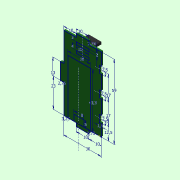
# Autodesk Inventor part: Motherboard_dummy
Saved by Autodesk Inventor 2015 (Build 190159000, 159)
## iProperties
Created: 2014-12-25
Part Number: Motherboard_dummy
Material: ABS Plastic
Document SubType Name: Modeling
Designer: Openlab
Density: 1.06 g/cm^3
Appearance: Smooth - Dark Forest Green
Mass: 9.08054 g
Surface Area: 59.127 cm^2
Volume: 8.56654 cm^3
Author: Openlab
Autodesk Inventor part; units mm, degrees
ref_plane "YZ Plane" through (0, 0, 0) normal (1, 0, 0) x (0, 1, 0)
ref_plane "XZ Plane" through (0, 0, 0) normal (0, 1, 0) x (-1, 0, 0)
ref_plane "XY Plane" through (0, 0, 0) normal (0, 0, 1) x (1, 0, 0)
sketch "Sketch1" plane through (0, 0, 0) normal (0, 1, 0) x (-1, 0, 0)
  line L0 (30, 0) -> (0, 0)
  line L1 (8.75, 0) -> (8.75, 43.3)
  line L2 (8.75, 43.3) -> (26.75, 43.3)
  line L3 (26.75, 43.3) -> (26.75, 0)
  line L4 (17.75, -19.2684) -> (17.75, 39.5149) construction
  line L5 (13.75, 5) -> (21.75, 5)
  line L6 (21.75, 5) -> (21.75, 0)
  line L7 (13.75, 0) -> (13.75, 5)
  line L8 (20, 56) -> (10, 56)
  line L9 (10, 56) -> (10, 54)
  line L10 (10, 54) -> (20, 54)
  line L11 (20, 54) -> (20, 56)
  line L12 (20, 50) -> (10, 50)
  line L13 (10, 50) -> (10, 48)
  line L14 (10, 48) -> (20, 48)
  line L15 (20, 48) -> (20, 50)
  line L16 (0, 9.5) -> (1.5, 9.5)
  line L17 (1.5, 9.5) -> (1.5, 15)
  line L18 (1.5, 15) -> (0, 15)
  line L19 (4.7373, 12.5) -> (-3.6899, 12.5) construction
  line L20 (0, 26.5) -> (1.5, 26.5)
  line L21 (1.5, 26.5) -> (1.5, 32)
  line L22 (1.5, 32) -> (0, 32)
  line L23 (5.7373, 29.5) -> (-2.6899, 29.5) construction
  line L24 (0, 43.5) -> (1.5, 43.5)
  line L25 (1.5, 43.5) -> (1.5, 49)
  line L26 (1.5, 49) -> (0, 49)
  line L27 (4.8698, 46.5) -> (-3.5573, 46.5) construction
  line L28 (10, 59) -> (10, 61.75)
  line L29 (10, 61.75) -> (20, 61.75)
  line L30 (20, 61.75) -> (20, 59)
  line L31 (15, 64.4653) -> (15, 46.4653) construction
  line L32 (0, 59) -> (10, 59)
  line L33 (20, 59) -> (30, 59)
  line L34 (0, 49) -> (0, 59)
  line L35 (0, 32) -> (0, 43.5)
  line L36 (0, 0) -> (0, 9.5)
  line L37 (0, 15) -> (0, 26.5)
  line L38 (30, 23) -> (32.75, 23)
  line L39 (32.75, 23) -> (32.75, 36)
  line L40 (32.75, 36) -> (30, 36)
  line L41 (30, 59) -> (30, 36)
  line L42 (30, 23) -> (30, 0)
  line L43 (10, 0) -> (10, -2.75)
  line L44 (10, -2.75) -> (20, -2.75)
  line L45 (20, -2.75) -> (20, 0)
  point P0 (17.75, 0)
  dimension "d47" = 18
  dimension "d49" = 43.3
  dimension "d50" = 5
  dimension "d51" = 8
  dimension "d52" = 30
  dimension "d53" = 59
  dimension "d106" = 10
  dimension "d107" = 2
  dimension "d109" = 4
  dimension "d112" = 12.5
  dimension "d113" = 2.5
  dimension "d114" = 3
  dimension "d116" = 2.5
  dimension "d117" = 3
  dimension "d118" = 2.5
  dimension "d119" = 3
  dimension "d120" = 17
  dimension "d121" = 17
  dimension "d123" = 10
  dimension "d125" = 1.5
  dimension "d126" = 2.75
  dimension "d127" = 3
  dimension "d128" = 23
  dimension "d129" = 13
  dimension "d130" = 2.75
  dimension "d131" = 3.25
  dimension "d132" = 10
  dimension "d134" = 10
  dimension "d135" = 10
  dimension "d136" = 2.75
  constraints: 92 end point, 34 perpendicular, 10 collinear, 8 horizontal, 6 point on line, 4 coincident, 4 parallel, 2 vertical, 1 horizontal alignment, 4 other
  measures "d47" distance of L2.start L2.end
  measures "d49" distance of L1.start L2.start
  measures "d50" distance of L7.start L5.start
  measures "d51" distance of L5.start L5.end
  measures "d52" distance of L0.start L0.end
  measures "d53" distance of L0.end L32.start
  measures "d106" distance of L10.end L9.end
  measures "d107" distance of L9.end L8.end
  measures "d109" distance between parallel lines of L12 L10
  measures "d112" distance between parallel lines of L0 L19
  measures "d113" distance between parallel lines of L19 L18
  measures "d114" distance between parallel lines of L16 L19
  measures "d116" distance between parallel lines of L23 L22
  measures "d117" distance between parallel lines of L20 L23
  measures "d118" distance between parallel lines of L27 L26
  measures "d119" distance between parallel lines of L24 L27
  measures "d120" distance between parallel lines of L19 L23
  measures "d121" distance between parallel lines of L23 L27
  measures "d123" distance of L28.end L29.end
  measures "d125" distance of L16.start L16.end
  measures "d126" distance of L28.start L28.end
  measures "d127" distance between parallel lines of L8 L33
  measures "d128" distance of L38.start L0.start
  measures "d129" distance of L38.end L39.end
  measures "d130" distance of L38.start L38.end
  measures "d131" distance between parallel lines of L42 L3
  measures "d132" distance of L30.end L33.end
  measures "d134" distance of L43.end L44.end
  measures "d135" horizontal distance of point (0, 0) L43.end
  measures "d136" distance of L43.start L43.end
extrude "Extrusion1" add sketch "Sketch1" along normal blind 1.5 contours L0 L3 L2 L1 L36 L16 L17 L18 L37 L20 L21 L22 L35 L24 L25 L26 L34 L32 L28 L29 L30 L33 L41 L40 L39 L38 L42 | L0 L6 L5 L7 L1 L2 L3 | L0 L7 L5 L6 | L45 L44 L43 L0 | L11 L10 L9 L8 | L15 L14 L13 L12
extrude "Extrusion2" add sketch "Sketch1" along normal blind 6 contours L0 L6 L5 L7 L1 L2 L3
sketch "Sketch2" plane through (0, 0, 0) normal (0, 0, -1) x (-1, 0, 0)
  line L0 (13.75, 10) -> (21.75, 10)
  line L1 (21.75, 10) -> (21.75, 6)
  line L2 (21.75, 6) -> (13.75, 6)
  line L3 (13.75, 6) -> (13.75, 10)
  line L4 (0, 0) -> (10, 0) projected
  line L5 (21.75, 6) -> (21.75, 10)
  point P0 (30, 0)
  dimension "d100" = 4
  dimension "d101" = 8
  constraints: 10 end point, 2 parallel, 1 collinear, 1 horizontal, 1 perpendicular
  measures "d100" distance of L2.end L0.start
  measures "d101" distance of L0.start L0.end
extrude "Extrusion7" add sketch "Sketch2" along normal blind 1.5
extrude "Extrusion8" add sketch "Sketch1" along normal blind 10 contours L11 L10 L9 L8 | L15 L14 L13 L12
extrude "Extrusion9" cut sketch "Sketch1" along normal blind 10 contours L0 L7 L5 L6
extrude "Extrusion10" add sketch "Sketch1" along normal blind 10 contours L0 L7 L5 L6
sketch "Sketch3" plane through (-1.5, 0, 49) normal (1, 0, 0) x (0, 0, -1)
  point P0 (49, 0)
body "Solid1"
